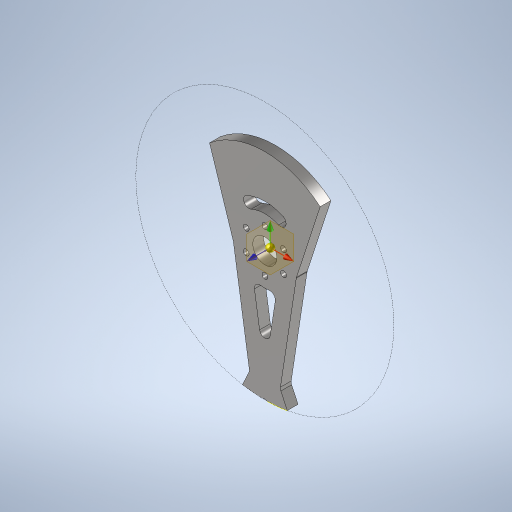
# Autodesk Inventor part: Blade (Bar 3)
Saved by Autodesk Inventor 2023.4 (Build 274418000, 418)
## iProperties
Created: 2022-10-17
Part Number: Blade (Bar 3)
Material: Steel, Alloy
Document SubType Name: Modeling
Designer: Nathan Cai
Density: 7.73 g/cm^3
Appearance: Semi-Polished
Mass: 199.695 g
Surface Area: 117.453 cm^2
Volume: 25.8337 cm^3
Author: Nathan Cai
Autodesk Inventor part; units mm, degrees
ref_plane "YZ Plane" through (0, 0, 0) normal (1, 0, 0) x (0, 1, 0)
ref_plane "XZ Plane" through (0, 0, 0) normal (0, 1, 0) x (-1, 0, 0)
ref_plane "XY Plane" through (0, 0, 0) normal (0, 0, 1) x (1, 0, 0)
sketch "Sketch1" plane through (0, 0, 0) normal (0, 0, 1) x (1, 0, 0)
  circle A0 centre (0, 0) radius 7.1437
  line L0 (0, 0) -> (0, 12.7) construction
  circle A1 centre (0, 12.7) radius 1.7526
  circle A2 centre (-10.9985, 6.35) radius 1.7526
  circle A3 centre (-10.9985, -6.35) radius 1.7526
  circle A4 centre (0, -12.7) radius 1.7526
  circle A5 centre (10.9985, -6.35) radius 1.7526
  circle A6 centre (10.9985, 6.35) radius 1.7526
  circle A7 centre (0, 0) radius 19.05
  circle A8 centre (0, 0) radius 76.2 construction
  line L1 (0, 0) -> (-13.232, -75.0424) construction
  line L2 (-13.232, -75.0424) -> (4.8119, -36.3472) construction
  line L3 (-13.232, -75.0424) -> (-9.0429, -66.0589)
  line L4 (-9.0429, -66.0589) -> (-18.8254, -2.9166)
  circle A9 centre (0, 0) radius 66.675 construction
  line L5 (0, 0) -> (0, -76.2) construction
  arc A10 (-13.232, -75.0424) -> (0, -76.2) centre (0, 0) ccw
  line L6 (13.232, -75.0424) -> (9.0429, -66.0589)
  line L7 (9.0429, -66.0589) -> (18.8254, -2.9166)
  arc A11 (0, -76.2) -> (13.232, -75.0424) centre (0, 0) ccw
  arc A12 (-2.5837, -18.874) -> (-6.1519, -22.5057) centre (-3.0143, -22.0196) ccw
  line L8 (-6.1519, -22.5057) -> (-3.1376, -41.9621)
  arc A13 (-3.1376, -41.9621) -> (0, -44.651) centre (0, -41.476) ccw
  arc A14 (6.1519, -22.5057) -> (2.5837, -18.874) centre (3.0143, -22.0196) ccw
  line L9 (6.1519, -22.5057) -> (3.1376, -41.9621)
  arc A15 (0, -44.651) -> (3.1376, -41.9621) centre (0, -41.476) ccw
  circle A16 centre (0, 0) radius 50.8 construction
  line L10 (-32.6536, 38.9151) -> (-18.1201, -5.8791)
  line L11 (-32.6536, 38.9151) -> (0, 0) construction
  arc A17 (0, 50.8) -> (-32.6536, 38.9151) centre (0, 0) ccw
  line L12 (32.6536, 38.9151) -> (18.1201, -5.8791)
  line L13 (32.6536, 38.9151) -> (0, 0) construction
  arc A18 (32.6536, 38.9151) -> (0, 50.8) centre (0, 0) ccw
  arc A19 (9.3927, 20.1427) -> (-9.3927, 20.1427) centre (0, 0) ccw construction
  arc A20 (10.7345, 23.0202) -> (-10.7345, 23.0202) centre (0, 0) ccw
  arc A21 (8.0509, 17.2652) -> (-8.0509, 17.2652) centre (0, 0) ccw
  arc A22 (8.0509, 17.2652) -> (10.7345, 23.0202) centre (9.3927, 20.1427) ccw
  arc A23 (-10.7345, 23.0202) -> (-8.0509, 17.2652) centre (-9.3927, 20.1427) ccw
  line L14 (-9.3927, 20.1427) -> (0, 0) construction
  line L15 (0, 0) -> (9.3927, 20.1427) construction
  line L16 (0, -72.9607) -> (-1.5036, -76.1852)
  line L17 (-1.5036, -76.1852) -> (0, -72.9607)
  line L18 (1.5036, -76.1852) -> (0, -72.9607)
  point P0 (-18.5915, -4.4261)
  point P1 (18.5915, -4.4261)
  point P2 (2.5837, -18.874)
  point P3 (-11.1375, -70.5506)
  point P4 (8.0509, 17.2652)
  point P5 (-8.0509, 17.2652)
  dimension "d10" = 133.35
  dimension "d0" = 14.2875
  dimension "d1" = 12.7
  dimension "d2" = 3.5052
  dimension "d5" = 360
  dimension "d7" = 38.1
  dimension "d8" = 152.4
  dimension "d9" = 15
  dimension "d11" = 10
  dimension "d12" = 6.35
  dimension "d14" = 6.35
  dimension "d15" = 9.525
  dimension "d16" = 101.6
  dimension "d17" = 80
  dimension "d18" = 50
  dimension "d19" = 3.175
  dimension "d20" = 22.225
  dimension "d25" = 11.1125
  constraints: 38 end point, 35 point on circle, 23 centre point, 10 tangent, 9 symmetric about line, 7 coincident, 4 point on line, 3 parallel, 2 concentric, 2 vertical, 1 collinear, 1 midpoint, 21 other
  measures "d0" diameter of A0
  measures "d1" distance of L0.start L0.end
  measures "d2" diameter of A1
  measures "d7" diameter of A7
  measures "d8" diameter of A8
  measures "d9" angle of L1 L2
  measures "d11" angle of L5 L1
  measures "d12" diameter of A12
  measures "d14" diameter of A13
  measures "d15" distance between parallel lines of L4 L8
  measures "d16" diameter of A16
  measures "d17" angle of L13 L11
  measures "d18" angle of L14 L15
  measures "d19" radius of A23
  measures "d20" radius of A19
  measures "d25" distance from line of point (-11.137, -70.551) L16
extrude "Extrusion1" add sketch "Sketch1" along normal blind 6.35 contours A7 | A7 A22 A20 A23 L4 L10 A17 A18 L12 L7 | L7 L12 A7 | L12 L7 L6 A11 L18 L16 A10 L3 L4 L10 A7 A12 L8 A13 A15 L9 A14 | A7 L10 L4
fillet "Fillet1" radius 3.175 5 edges at (18.5915, -4.4261, 3.175) (9.0429, -66.0589, 3.175) (-18.5915, -4.4261, 3.175) (-9.0429, -66.0589, 3.175) (0, -72.9607, 3.175)
sketch "Sketch2" plane through (0, 0, 6.35) normal (0, 0, 1) x (1, 0, 0)
  arc A0 (1.5036, -76.1852) -> (13.232, -75.0424) centre (0, 0) ccw projected
  circle A1 centre (0, 0) radius 76.2 construction
  constraints: 1 coincident, 3 other
body "Solid1"
